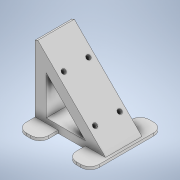
# Autodesk Inventor part: Gravitational viscometer P2
Saved by Autodesk Inventor 2020 (Build 240168000, 168)
## iProperties
Created: 2023-07-29
Part Number: Gravitational viscometer P2
Material: Generic
Document SubType Name: Modeling
Designer: 56992
Density: 1 g/cm^3
Appearance: Default
Author: 56992
Autodesk Inventor part; units mm, degrees
ref_plane "YZ Plane" through (0, 0, 0) normal (1, 0, 0) x (0, 1, 0)
ref_plane "XZ Plane" through (0, 0, 0) normal (0, 1, 0) x (-1, 0, 0)
ref_plane "XY Plane" through (0, 0, 0) normal (0, 0, 1) x (1, 0, 0)
sketch "Sketch1" plane through (0, 0, 0) normal (0, 0, 1) x (1, 0, 0)
  line L0 (0, 0) -> (80, 0)
  line L1 (80, 0) -> (80, 80)
  line L2 (80, 80) -> (0, 80)
  line L3 (0, 80) -> (0, 0)
  line L4 (80, 0) -> (0, 80)
  dimension "d0" = 80
  dimension "d1" = 80
  dimension "d2" = 45
  constraints: 10 end point, 2 parallel, 1 horizontal, 1 perpendicular, 1 point on line
  measures "d0" distance between parallel lines of L0 L2
  measures "d1" distance between parallel lines of L3 L1
  measures "d2" angle of L0 L4
extrude "Extrusion1" add sketch "Sketch1" against normal blind 40 contours L3 L4 L0
sketch "Sketch2" plane through (80, 0, -40) normal (0.7071, 0.7071, 0) x (-0.7071, 0.7071, 0)
  circle A0 centre (78.1371, 33.5) radius 2.1
  circle A1 centre (78.1371, 6.5) radius 2.1
  line L0 (0, 40) -> (113.1371, 40) projected
  line L1 (113.1371, 0) -> (0, 0) projected
  circle A2 centre (29.6371, 33.5) radius 2.1
  circle A3 centre (29.6371, 6.5) radius 2.1
  line L2 (113.1371, 40) -> (113.1371, 0) projected
  point P0 (56.5685, 40)
  dimension "d5" = 27
  dimension "d6" = 4.2
  dimension "d7" = 4.2
  dimension "d8" = 6.5
  dimension "d10" = 27
  dimension "d11" = 4.2
  dimension "d12" = 4.2
  dimension "d13" = 48.5
  dimension "d29" = 35
  dimension "d30" = 35
  dimension "d31" = 48.5
  dimension "d32" = 6.5
  constraints: 4 centre point
  measures "d5" distance of A0.centre A1.centre
  measures "d6" diameter of A0
  measures "d7" diameter of A1
  measures "d8" distance from line of L0 A0.centre
  measures "d10" distance of A3.centre A2.centre
  measures "d11" diameter of A2
  measures "d12" diameter of A3
  measures "d13" distance of A3.centre A1.centre
  measures "d29" distance from line of L2 A1.centre
  measures "d30" distance from line of L2 A0.centre
  measures "d31" distance of A0.centre A2.centre
  measures "d32" distance from line of L0 A2.centre
extrude "Extrusion2" cut sketch "Sketch2" against normal blind 10
fillet "Fillet1" radius 0.4 4 edges at (26.2337, 53.7663, -33.5) (26.2337, 53.7663, -6.5) (60.5283, 19.4717, -6.5) (60.5283, 19.4717, -33.5)
sketch "Sketch3" plane through (0, 0, -40) normal (0, 0, -1) x (-1, 0, 0)
  line L0 (0, 80) -> (-80, 0) projected
  line L1 (0, 0) -> (0, 80) projected
  line L2 (-80, 0) -> (0, 80)
  line L3 (0, 80) -> (0, 0)
  line L4 (0, 0) -> (-80, 0)
  line L5 (-91.5147, -28.4853) -> (-12, 51.0294)
  line L6 (-12, 51.0294) -> (-12, 0)
  line L7 (-12, 8) -> (-55.0294, 8)
  dimension "d17" = 12
  dimension "d18" = 8
  constraints: 12 end point, 2 point on line, 1 collinear, 1 horizontal, 1 perpendicular, 1 other
  measures "d17" distance between parallel lines of L1 L6
  measures "d18" distance between parallel lines of L4 L7
extrude "Extrusion3" cut sketch "Sketch3" against normal blind 40 contours L5 L6 L7
sketch "Sketch4" plane through (0, 0, 0) normal (0, -1, 0) x (1, 0, 0)
  line L0 (-20, -60) -> (80, -60)
  line L1 (80, -60) -> (80, 20)
  line L2 (80, 20) -> (-20, 20)
  line L3 (-20, 20) -> (-20, -60)
  line L4 (80, 0) -> (80, -40) projected
  line L5 (80, -40) -> (0, -40) projected
  line L6 (0, 0) -> (80, 0) projected
  line L7 (50, 20) -> (10, 20)
  line L8 (10, 20) -> (10, -60)
  line L9 (10, -60) -> (50, -60)
  line L10 (50, -60) -> (50, 20)
  point P0 (10, 0)
  point P1 (10, 20)
  point P2 (10, -40)
  point P3 (50, -40)
  point P4 (50, 0)
  dimension "d21" = 100
  dimension "d22" = 0
  dimension "d23" = 20
  dimension "d24" = 20
  dimension "d25" = 30
  dimension "d26" = 30
  constraints: 14 end point, 3 parallel, 2 horizontal, 2 perpendicular, 2 point on line, 1 vertical, 3 other
  measures "d22" distance between parallel lines of L4 L1
  measures "d23" distance between parallel lines of L5 L0
  measures "d24" distance between parallel lines of L6 L2
  measures "d25" distance between parallel lines of L1 L10
extrude "Extrusion4" [suppressed]
chamfer "Chamfer1" distance 4 angle 45 1 edges at (0, 80, -20)
fillet "Fillet2" [suppressed]
sketch "Sketch5" plane through (0, 0, 0) normal (0, -1, 0) x (1, 0, 0)
  line L0 (0, 20) -> (80, 20)
  line L1 (80, 20) -> (80, -60)
  line L2 (80, -60) -> (0, -60)
  line L3 (0, -60) -> (0, 20)
  line L4 (0, 0) -> (80, 0) projected
  line L5 (80, -40) -> (0, -40) projected
  line L6 (80, 0) -> (80, -40) projected
  line L7 (25, 20) -> (55, 20)
  line L8 (55, 20) -> (55, -60)
  line L9 (55, -60) -> (25, -60)
  line L10 (25, -60) -> (25, 20)
  dimension "d37" = 20
  dimension "d38" = 20
  dimension "d39" = 0
  dimension "d40" = 80
  dimension "d41" = 25
  dimension "d42" = 25
  constraints: 16 end point, 4 parallel, 2 horizontal, 2 perpendicular, 2 point on line
  measures "d37" distance between parallel lines of L4 L0
  measures "d38" distance between parallel lines of L5 L2
  measures "d39" distance between parallel lines of L6 L1
  measures "d40" distance between parallel lines of L1 L3
  measures "d41" distance between parallel lines of L3 L10
  measures "d42" distance between parallel lines of L1 L8
extrude "Extrusion5" add sketch "Sketch5" against normal blind 3 contours L0 L10 L4 L3 | L4 L10 L5 L3 | L0 L1 L4 L8 | L5 L10 L2 L3 | L4 L1 L5 L8 | L5 L1 L2 L8
fillet "Fillet3" radius 10 8 edges at (25, 1.5, 20) (0, 1.5, 20) (55, 1.5, 20) (80, 1.5, 20) (80, 1.5, -60) (55, 1.5, -60) (25, 1.5, -60) (0, 1.5, -60)
body "Solid1"
